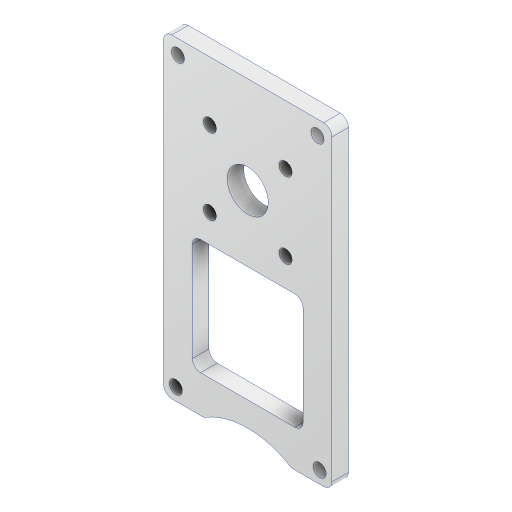
# Autodesk Inventor part: 링크2고정부
Saved by Autodesk Inventor 2023.2 (Build 272271000, 271)
## iProperties
Created: 2022-01-25
Part Number: 링크2고정부
Material: 알루미늄 6061
Document SubType Name: Modeling
Designer: BAEK
Density: 2.7 g/cm^3
Appearance: 알루미늄 - 평지
Mass: 23.6272 g
Surface Area: 61.7806 cm^2
Volume: 8.7508 cm^3
Author: BAEK
Autodesk Inventor part; units mm, degrees
ref_plane "YZ Plane" through (0, 0, 0) normal (1, 0, 0) x (0, 1, 0)
ref_plane "XZ Plane" through (0, 0, 0) normal (0, 1, 0) x (-1, 0, 0)
ref_plane "XY Plane" through (0, 0, 0) normal (0, 0, 1) x (1, 0, 0)
sketch "스케치1" plane through (0, 0, 0) normal (0, 0, 1) x (1, 0, 0)
  line L0 (28.124, 3.5) -> (28.124, -58.5)
  line L1 (-12.7588, 3.5) -> (-12.7588, -58.5)
  line L2 (-12.7588, -58.5) -> (28.124, -58.5)
  line L3 (-12.7588, 3.5) -> (-12.7588, 4.4)
  line L4 (28.124, 4.4) -> (28.124, 3.5)
  line L5 (-12.7588, 4.4) -> (-12.7588, 10)
  line L6 (-12.7588, 10) -> (28.124, 10)
  line L7 (28.124, 10) -> (28.124, 4.4)
  dimension "d16" = 68.5
  dimension "d50" = 40.8828
  constraints: 16 end point, 3 vertical, 2 horizontal, 1 perpendicular
  measures "d16" distance between parallel lines of L2 L6
  measures "d50" distance of L5.end L6.end
extrude "돌출2" add sketch "스케치1" along normal blind 4
sketch "스케치4" plane through (0, 0, 4) normal (0, 0, 1) x (1, 0, 0)
  circle A0 centre (7.6826, -9.5) radius 5
  point P0 (0, 0)
  constraints: 1 centre point
sketch "스케치6" plane through (0, 0, 4) normal (0, 0, 1) x (1, 0, 0)
  circle A0 centre (7.6826, -9.5) radius 13 construction
  line L0 (7.6826, -9.5) -> (-1.5098, -0.3076) construction
  line L1 (7.6826, -9.5) -> (20.6826, -9.5) construction
  line L2 (7.6826, -9.5) -> (-1.5098, -18.6924) construction
  line L3 (7.6826, -9.5) -> (20.6826, -9.5) construction
  circle A1 centre (-1.5098, -0.3076) radius 1.6
  circle A2 centre (-1.5098, -18.6924) radius 1.6
  circle A3 centre (7.6826, -9.5) radius 5 projected
  circle A4 centre (16.875, -0.3076) radius 1.6
  line L4 (7.6826, -9.5) -> (16.875, -18.6924) construction
  circle A5 centre (16.875, -18.6924) radius 1.6
  point P0 (0, 0)
  dimension "d51" = 26
  dimension "d52" = 135
  dimension "d53" = 135
  dimension "d54" = 3.2
  dimension "d55" = 3.2
  dimension "d56" = 3.2
  dimension "d57" = 3.2
  constraints: 10 end point, 5 centre point, 4 coincident, 4 point on circle, 2 equal length, 2 horizontal, 2 point on line
  measures "d51" diameter of A0
  measures "d52" angle of L1 L0
  measures "d53" angle of L2 L3
  measures "d54" diameter of A1
  measures "d55" diameter of A2
  measures "d56" diameter of A4
  measures "d57" diameter of A5
extrude "돌출4" cut sketch "스케치6" against normal up to surface (4 mm away)
sketch "스케치5" plane through (0, 0, 4) normal (0, 0, 1) x (1, 0, 0)
  line L0 (-12.7588, 10) -> (-12.7588, -58.5) projected
  line L1 (-12.7588, -58.5) -> (28.124, -58.5) projected
  line L2 (28.124, -58.5) -> (28.124, 10) projected
  line L3 (28.124, 10) -> (-12.7588, 10) projected
  circle A0 centre (-9.7588, -59.5) radius 1.6
  circle A1 centre (25.124, -59.5) radius 1.6
  circle A2 centre (-9.2588, 10.5) radius 1.6
  circle A3 centre (24.624, 10.5) radius 1.6
  line L4 (28.124, 10) -> (28.124, 14)
  line L5 (28.124, -58.5) -> (28.124, 10) projected
  line L6 (28.124, -58.5) -> (28.124, -62.5)
  point P0 (0, 0)
  dimension "d36" = 3.2
  dimension "d37" = 3.2
  dimension "d38" = 3.2
  dimension "d39" = 3.2
  dimension "d40" = 3
  dimension "d42" = 3.5
  dimension "d44" = 3.5
  dimension "d46" = 3
  dimension "d64" = 4
  dimension "d65" = 3.5
  dimension "d66" = 3.5
  dimension "d67" = 4
  dimension "d68" = 3
  dimension "d69" = 3
  constraints: 4 centre point, 4 end point, 1 point on line, 1 vertical
  measures "d36" diameter of A0
  measures "d37" diameter of A1
  measures "d38" diameter of A2
  measures "d39" diameter of A3
  measures "d40" distance from line of L0 A0.centre
  measures "d42" distance from line of L0 A2.centre
  measures "d44" distance from line of L2 A3.centre
  measures "d46" distance from line of L2 A1.centre
  measures "d64" distance of L2.end L4.end
  measures "d65" horizontal distance of L4.end A3.centre
  measures "d66" vertical distance of L4.end A2.centre
  measures "d67" distance of L1.end L6.end
  measures "d68" horizontal distance of L6.end A1.centre
  measures "d69" vertical distance of A0.centre L6.end
extrude "돌출3" cut sketch "스케치5" against normal up to surface (4 mm away) contours A2 L3 | L3 A2 | A0 L1 | L1 A0 | A3 L3 | L3 A3 | A1 L1 | L1 A1
sketch "스케치7" plane through (0, 0, 4) normal (0, 0, 1) x (1, 0, 0)
  line L0 (-12.7588, 10) -> (-12.7588, 14)
  arc A0 (23.1041, 10) -> (26.1439, 10) centre (24.624, 10.5) ccw projected
  arc A1 (26.373, -58.5) -> (23.875, -58.5) centre (25.124, -59.5) ccw projected
  arc A2 (-10.7787, 10) -> (-7.7389, 10) centre (-9.2588, 10.5) ccw projected
  arc A3 (-8.5098, -58.5) -> (-11.0078, -58.5) centre (-9.7588, -59.5) ccw projected
  circle A4 centre (16.875, -0.3076) radius 1.6 projected
  circle A5 centre (-1.5098, -18.6924) radius 1.6 projected
  circle A6 centre (7.6826, -9.5) radius 5 projected
  circle A7 centre (16.875, -18.6924) radius 1.6 projected
  circle A8 centre (-1.5098, -0.3076) radius 1.6 projected
  line L1 (-12.7588, -58.5) -> (-11.0078, -58.5) projected
  line L2 (28.124, -58.5) -> (28.124, 10) projected
  line L3 (28.124, 10) -> (26.1439, 10) projected
  line L4 (-12.7588, 10) -> (-12.7588, -58.5) projected
  line L5 (28.124, 10) -> (28.124, 14)
  line L6 (28.124, 14) -> (-12.7588, 14)
  line L7 (28.124, -58.5) -> (28.124, 10) projected
  line L8 (-12.7588, -58.5) -> (28.124, -58.5) projected
  line L9 (28.124, -58.5) -> (-12.7588, -58.5)
  line L10 (-12.7588, -58.5) -> (-12.7588, -62.5)
  line L11 (-12.7588, -62.5) -> (28.124, -62.5)
  line L12 (28.124, -62.5) -> (28.124, -58.5)
  line L13 (23.1041, 10) -> (-7.7389, 10) projected
  line L14 (-10.7787, 10) -> (-12.7588, 10) projected
  line L15 (-8.5098, -58.5) -> (23.875, -58.5) projected
  line L16 (26.373, -58.5) -> (28.124, -58.5) projected
  circle A9 centre (24.624, 10.5) radius 1.6
  arc A10 (-10.7787, 10) -> (-7.7389, 10) centre (-9.2588, 10.5) ccw projected
  circle A11 centre (-9.2588, 10.5) radius 1.6
  circle A12 centre (25.124, -59.5) radius 1.6
  arc A13 (-8.5098, -58.5) -> (-11.0078, -58.5) centre (-9.7588, -59.5) ccw projected
  circle A14 centre (-9.7588, -59.5) radius 1.6
  point P0 (0, 0)
  point P1 (26.373, -58.5)
  point P2 (23.875, -58.5)
  point P3 (-7.7389, 10)
  dimension "d60" = 4
  dimension "d61" = 4
  constraints: 14 end point, 4 centre point, 4 coincident, 4 perpendicular, 2 vertical, 1 concentric, 1 horizontal, 1 point on line
  measures "d60" distance of L0.start L0.end
  measures "d61" distance of L1.start L10.end
extrude "돌출6" add sketch "스케치7" against normal up to surface (4 mm away) contours L0 L6 L5 L3 A9 L13 A11 L14 | L1 A14 L8 A12 L12 L11 L10
fillet "모깎기3" radius 2 4 edges at (28.124, 14, 2) (-12.7588, 14, 2) (-12.7588, -62.5, 2) (28.124, -62.5, 2)
sketch "스케치10" plane through (0, 0, 4) normal (0, 0, 1) x (1, 0, 0)
  line L0 (-3.7588, -53.5) -> (19.124, -53.5)
  line L1 (21.124, -51.5) -> (21.124, -27.5)
  line L2 (19.124, -25.5) -> (-3.7588, -25.5)
  line L3 (-5.7588, -27.5) -> (-5.7588, -51.5)
  circle A0 centre (-9.7588, -59.5) radius 1.6 projected
  line L4 (28.124, -60.5) -> (28.124, 12) projected
  line L5 (-12.7588, 12) -> (-12.7588, -60.5) projected
  circle A1 centre (25.124, -59.5) radius 1.6 projected
  circle A2 centre (24.624, 10.5) radius 1.6 projected
  circle A3 centre (-9.2588, 10.5) radius 1.6 projected
  circle A4 centre (16.875, -0.3076) radius 1.6 projected
  circle A5 centre (-1.5098, -18.6924) radius 1.6 projected
  circle A6 centre (7.6826, -9.5) radius 5 projected
  circle A7 centre (16.875, -18.6924) radius 1.6 projected
  circle A8 centre (-1.5098, -0.3076) radius 1.6 projected
  arc A9 (-5.7588, -51.5) -> (-3.7588, -53.5) centre (-3.7588, -51.5) ccw
  arc A10 (19.124, -53.5) -> (21.124, -51.5) centre (19.124, -51.5) ccw
  arc A11 (21.124, -27.5) -> (19.124, -25.5) centre (19.124, -27.5) ccw
  arc A12 (-3.7588, -25.5) -> (-5.7588, -27.5) centre (-3.7588, -27.5) ccw
  arc A13 (26.124, -62.5) -> (28.124, -60.5) centre (26.124, -60.5) ccw projected
  arc A14 (28.124, 12) -> (26.124, 14) centre (26.124, 12) ccw projected
  line L6 (26.124, 14) -> (-10.7588, 14) projected
  arc A15 (-10.7588, 14) -> (-12.7588, 12) centre (-10.7588, 12) ccw projected
  arc A16 (-12.7588, -60.5) -> (-10.7588, -62.5) centre (-10.7588, -60.5) ccw projected
  line L7 (-10.7588, -62.5) -> (26.124, -62.5) projected
  point P0 (0, 0)
  point P1 (-5.7588, -53.5)
  point P2 (21.124, -25.5)
  point P3 (21.124, -53.5)
  point P4 (-5.7588, -25.5)
  dimension "d84" = 16
  dimension "d87" = 7
  dimension "d88" = 7
  dimension "d89" = 2
  constraints: 8 end point, 8 point on circle, 8 point on line, 8 tangent, 4 centre point, 3 equal radius, 2 parallel, 1 horizontal, 1 perpendicular
  measures "d84" distance from line of A6.centre L2
  measures "d87" distance between parallel lines of L5 L3
  measures "d88" distance between parallel lines of L4 L1
  measures "d89" radius of A9
extrude "돌출7" cut sketch "스케치10" against normal up to surface (4 mm away) contours A9 L3 A12 L2 A11 L1 A10 L0
sketch "스케치11" plane through (0, 0, 4) normal (0, 0, 1) x (1, 0, 0)
  line L0 (-10.7588, 14) -> (26.124, 14) projected
  line L1 (7.6826, 14) -> (7.6826, -136) construction
  circle A0 centre (7.6826, -79.433) radius 20
  arc A1 (21.124, -27.5) -> (19.124, -25.5) centre (19.124, -27.5) ccw projected
  line L2 (21.124, -27.5) -> (21.124, -51.5) projected
  arc A2 (19.124, -53.5) -> (21.124, -51.5) centre (19.124, -51.5) ccw projected
  line L3 (19.124, -53.5) -> (-3.7588, -53.5) projected
  arc A3 (-5.7588, -51.5) -> (-3.7588, -53.5) centre (-3.7588, -51.5) ccw projected
  line L4 (-5.7588, -51.5) -> (-5.7588, -27.5) projected
  arc A4 (-3.7588, -25.5) -> (-5.7588, -27.5) centre (-3.7588, -27.5) ccw projected
  line L5 (-3.7588, -25.5) -> (19.124, -25.5) projected
  circle A5 centre (25.124, -59.5) radius 1.6 projected
  circle A6 centre (-9.7588, -59.5) radius 1.6 projected
  line L6 (28.124, -60.5) -> (28.124, 12) projected
  line L7 (-12.7588, 12) -> (-12.7588, -60.5) projected
  circle A7 centre (24.624, 10.5) radius 1.6 projected
  circle A8 centre (-9.2588, 10.5) radius 1.6 projected
  circle A9 centre (16.875, -0.3076) radius 1.6 projected
  circle A10 centre (-1.5098, -18.6924) radius 1.6 projected
  circle A11 centre (7.6826, -9.5) radius 5 projected
  circle A12 centre (16.875, -18.6924) radius 1.6 projected
  circle A13 centre (-1.5098, -0.3076) radius 1.6 projected
  arc A14 (26.124, -62.5) -> (28.124, -60.5) centre (26.124, -60.5) ccw projected
  arc A15 (28.124, 12) -> (26.124, 14) centre (26.124, 12) ccw projected
  line L8 (26.124, 14) -> (-10.7588, 14) projected
  arc A16 (-10.7588, 14) -> (-12.7588, 12) centre (-10.7588, 12) ccw projected
  arc A17 (-12.7588, -60.5) -> (-10.7588, -62.5) centre (-10.7588, -60.5) ccw projected
  line L9 (-10.7588, -62.5) -> (26.124, -62.5) projected
  point P0 (0, 0)
  point P1 (-2.9604, -62.5)
  point P2 (18.3256, -62.5)
  dimension "d90" = 150
  dimension "d91" = 40
  dimension "d92" = 25.933
  constraints: 2 end point, 1 centre point, 1 midpoint, 1 point on line, 1 vertical
  measures "d90" distance of L1.start L1.end
  measures "d91" diameter of A0
  measures "d92" distance from line of L3 A0.centre
extrude "돌출8" cut sketch "스케치11" against normal up to surface (4 mm away) contours A0 L9 picked at (6.936, -61.5196)
